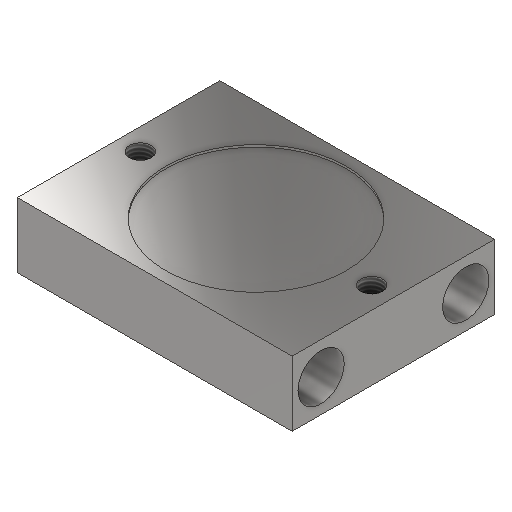
# Autodesk Inventor part: HayashiProbeHead_sub
Saved by Autodesk Inventor 2026.2 (Build 302298000, 298)
## iProperties
Created: 2026-08-31
Part Number: HayashiProbeHead_sub
Material: ステンレス鋼 440C
Document SubType Name: Modeling
Designer: zetsu
Density: 7.75 g/cm^3
Appearance: 半つや出し
Author: zetsu
Autodesk Inventor part; units mm, degrees
ref_plane "YZ Plane" through (0, 0, 0) normal (1, 0, 0) x (0, 1, 0)
ref_plane "XZ Plane" through (0, 0, 0) normal (0, 1, 0) x (-1, 0, 0)
ref_plane "XY Plane" through (0, 0, 0) normal (0, 0, 1) x (1, 0, 0)
sketch "スケッチ1" plane through (0, 0, 0) normal (0, 1, 0) x (-1, 0, 0)
  line L0 (19, -14) -> (-19, -14)
  line L1 (-19, -14) -> (-19, 14)
  line L2 (-19, 14) -> (19, 14)
  line L3 (19, 14) -> (19, -14)
  line L4 (0, -29.0161) -> (0, 0) construction
  line L5 (0, 0) -> (-35.7009, 0) construction
  dimension "d0" = 28
  dimension "d1" = 38
  constraints: 12 end point, 2 parallel, 2 perpendicular, 1 horizontal, 1 vertical, 2 other
  measures "d0" distance of L2.end L0.start
  measures "d1" distance of L1.end L2.end
extrude "押し出し1" add sketch "スケッチ1" along normal blind 9
sketch "スケッチ2" plane through (19, 0, 14) normal (1, 0, 0) x (0, 0, -1)
  circle A0 centre (4, 4.5) radius 3.2
  circle A1 centre (24, 4.5) radius 3.2
  line L0 (14, 0) -> (14, 13.3694) construction
  line L1 (0, 0) -> (28, 0) projected
  dimension "d4" = 6.4
  dimension "d5" = 6.4
  dimension "d6" = 20
  dimension "d7" = 4.5
  constraints: 2 centre point, 2 end point, 1 symmetric about line, 1 vertical
  measures "d4" diameter of A0
  measures "d5" diameter of A1
  measures "d6" distance of A1.centre A0.centre
  measures "d7" distance from line of L1 A0.centre
extrude "押し出し2" cut sketch "スケッチ2" against normal through all
sketch "スケッチ3" plane through (0, 9, 0) normal (0, 1, 0) x (1, 0, 0)
  circle A0 centre (0, 0) radius 12.5
  dimension "d10" = 25
  constraints: 1 centre point, 1 coincident
  measures "d10" diameter of A0
extrude "押し出し3" cut sketch "スケッチ3" against normal blind 0.3
sketch "スケッチ4" plane through (0, 9, 0) normal (0, 1, 0) x (1, 0, 0)
  circle A0 centre (-16, 0) radius 1.5
  circle A1 centre (16, 0) radius 1.5
  line L0 (-19, 14) -> (-19, -14) projected
  line L1 (19, -14) -> (19, 14) projected
  point P0 (0, 0)
  dimension "d13" = 3
  dimension "d14" = 3
  dimension "d15" = 3
  dimension "d16" = 3
  constraints: 2 centre point
  measures "d13" diameter of A0
  measures "d14" diameter of A1
  measures "d15" distance from line of L0 A0.centre
  measures "d16" distance from line of L1 A1.centre
extrude "押し出し4" cut sketch "スケッチ4" against normal through all
thread "ねじ1" size "M3x0.5" class "6H" standard "ANSI Metric M Profile" full length
thread "ねじ2" size "M3x0.5" class "6H" standard "ANSI Metric M Profile" full length
